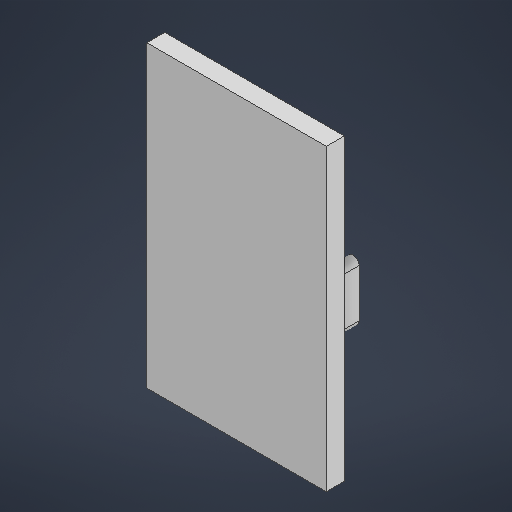
# Autodesk Inventor part: motor box
Saved by Autodesk Inventor 2026.2 (Build 302298010, 298A)
## iProperties
Created: 2026-03-04
Part Number: motor box
Material: Generic
Document SubType Name: Modeling
Designer: shahd
Density: 1 g/cm^3
Appearance: Default
Author: shahd
Autodesk Inventor part; units mm, degrees
ref_plane "YZ Plane" through (0, 0, 0) normal (1, 0, 0) x (0, 1, 0)
ref_plane "XZ Plane" through (0, 0, 0) normal (0, 1, 0) x (-1, 0, 0)
sketch "Sketch1" plane through (0, 0, 0) normal (0, 0, 1) x (1, 0, 0)
  line L0 (0, 0) -> (30, 0)
  line L1 (30, 0) -> (30, 50)
  line L2 (30, 50) -> (0, 50)
  line L3 (0, 50) -> (0, 0)
  dimension "d0" = 30
  dimension "d1" = 50
  constraints: 8 end point, 2 parallel, 1 horizontal, 1 perpendicular
  measures "d0" distance of L2.end L1.end
  measures "d1" distance of L1.end L0.end
extrude "Extrusion1" add sketch "Sketch1" along normal blind 3
ref_plane "Work Plane1" through (15, 0, 0) normal (1, 0, 0) x (0, 0, -1)
sketch "Sketch4" plane through (0, 0, 0) normal (0, 0, -1) x (-1, 0, 0)
  line L0 (-28, 30) -> (-28, 20) construction
  line L1 (-29, 29) -> (-29, 21)
  line L2 (-27, 21) -> (-27, 29)
  arc A0 (-27, 29) -> (-29, 29) centre (-28, 29) ccw
  arc A1 (-29, 21) -> (-27, 21) centre (-28, 21) ccw
  line L3 (-2, 30) -> (-2, 20) construction
  line L4 (-3, 29) -> (-3, 21)
  line L5 (-1, 21) -> (-1, 29)
  arc A2 (-1, 29) -> (-3, 29) centre (-2, 29) ccw
  arc A3 (-3, 21) -> (-1, 21) centre (-2, 21) ccw
  line L6 (-30, 0) -> (-30, 50) projected
  point P0 (0, 0)
  point P1 (-28, 25)
  point P2 (-2, 25)
  dimension "d19" = 25
  dimension "d20" = 1
  dimension "d21" = 1
  dimension "d22" = 10
  dimension "d23" = 10
  dimension "d25" = 1
  dimension "d29" = 1
  constraints: 16 end point, 16 point on circle, 8 tangent, 4 centre point, 4 point on line, 3 parallel, 2 midpoint, 1 horizontal alignment, 1 vertical
  measures "d19" vertical distance of point (0, 0) point (-2, 25)
  measures "d20" radius of A0
  measures "d21" radius of A2
  measures "d22" distance of point (-28, 20) point (-28, 30)
  measures "d23" distance of point (-2, 20) point (-2, 30)
  measures "d25" distance from line of point (0, 0) L5
  measures "d29" distance between parallel lines of L6 L1
extrude "Extrusion4" add sketch "Sketch4" along normal blind 3.5
body "Solid1"
